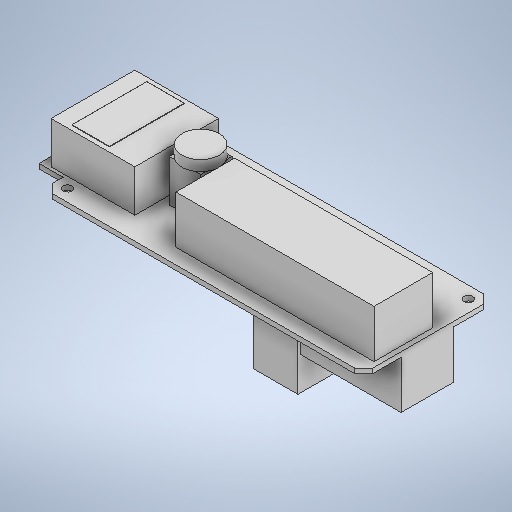
# Autodesk Inventor part: teaser_PCB
Saved by Autodesk Inventor 2025.2 (Build 292293000, 293)
## iProperties
Created: 2025-03-24
Part Number: teaser_PCB
Material: Generic
Document SubType Name: Modeling
Designer: Acer
Density: 1 g/cm^3
Appearance: Default
Author: Acer
Autodesk Inventor part; units mm, degrees
ref_plane "YZ Plane" through (0, 0, 0) normal (1, 0, 0) x (0, 1, 0)
ref_plane "XZ Plane" through (0, 0, 0) normal (0, 1, 0) x (-1, 0, 0)
ref_plane "XY Plane" through (0, 0, 0) normal (0, 0, 1) x (1, 0, 0)
sketch "Sketch1" plane through (0, 0, 0) normal (0, 1, 0) x (-1, 0, 0)
  line L0 (-57.5, 21.5) -> (57.5, 21.5)
  line L1 (57.5, 21.5) -> (57.5, -21.5)
  line L2 (57.5, -21.5) -> (-57.5, -21.5)
  line L3 (-57.5, -21.5) -> (-57.5, 21.5)
  line L4 (-57.5, 21.5) -> (57.5, -21.5) construction
  line L5 (57.5, 21.5) -> (-57.5, -21.5) construction
  point P0 (0, 0)
  dimension "d0" = 115
  dimension "d1" = 43
  constraints: 12 end point, 2 midpoint, 2 parallel, 1 horizontal, 1 perpendicular
  measures "d0" distance of L1.end L2.end
  measures "d1" distance of L0.end L1.end
extrude "Extrusion1" add sketch "Sketch1" along normal blind 1.6
sketch "Sketch2" plane through (0, 1.6, 0) normal (0, 1, 0) x (1, 0, 0)
  line L0 (57.5, 21.5) -> (-57.5, 21.5) projected
  line L1 (57.5, 21.5) -> (54.5, 21.5)
  line L2 (57.5, -21.5) -> (57.5, 21.5) projected
  line L3 (54.5, 21.5) -> (57.5, 21.5)
  line L4 (57.5, 21.5) -> (57.5, 18.5)
  line L5 (57.5, 18.5) -> (54.5, 21.5)
  point P0 (0, 0)
  dimension "d4" = 3
  dimension "d5" = 3
  constraints: 8 end point, 2 point on line, 1 perpendicular
  measures "d4" distance of L0.start L1.end
  measures "d5" distance of L0.start L4.end
extrude "Extrusion2" cut sketch "Sketch2" against normal blind 1.6
sketch "Sketch3" plane through (0, 1.6, 0) normal (0, 1, 0) x (1, 0, 0)
  line L0 (57.5, -21.5) -> (57.5, 18.5) projected
  circle A0 centre (53.5, 17.5) radius 1.5
  point P0 (0, 0)
  dimension "d11" = 3
  constraints: 1 centre point
  measures "d11" diameter of A0
extrude "Extrusion3" cut sketch "Sketch3" against normal blind 1.6
sketch "Sketch4" plane through (0, 1.6, 0) normal (0, 1, 0) x (1, 0, 0)
  line L0 (-57.5, 21.5) -> (-57.5, -21.5) projected
  line L1 (-57.5, 15) -> (-49.5, 15)
  line L2 (-49.5, 15) -> (-49.5, 18.5)
  line L3 (54.5, 21.5) -> (-57.5, 21.5) projected
  line L4 (-46.5, 21.5) -> (-49.5, 18.5)
  circle A0 centre (-45.5, 18) radius 1.5
  point P0 (0, 0)
  dimension "d15" = 8
  dimension "d16" = 3.5
  dimension "d20" = 3
  constraints: 6 end point, 1 centre point, 1 perpendicular, 1 point on line
  measures "d15" distance of L1.start L1.end
  measures "d16" distance of L1.end L2.end
  measures "d20" diameter of A0
extrude "Extrusion4" cut sketch "Sketch4" against normal blind 1.6 contours L3 L4 L2 L1 L0
sketch "Sketch5" plane through (0, 1.6, 0) normal (0, 1, 0) x (1, 0, 0)
  line L0 (54.5, 21.5) -> (-46.5, 21.5) projected
  circle A0 centre (-45.5, 17.5) radius 1.5
  point P0 (0, 0)
  dimension "d25" = 3
  constraints: 1 centre point
  measures "d25" diameter of A0
extrude "Extrusion5" cut sketch "Sketch5" against normal blind 1.6
mirror "Mirror1" about plane through (0, 0, 0) normal (0, 0, 1) of "Extrusion4", "Extrusion5", "Extrusion2"
sketch "Sketch7" plane through (0, 1.6, 0) normal (0, 1, 0) x (1, 0, 0)
  line L0 (-54.4988, 14.0073) -> (-26.4988, 14.0073)
  line L1 (-26.4988, 14.0073) -> (-26.4988, -13.9927)
  line L2 (-26.4988, -13.9927) -> (-54.4988, -13.9927)
  line L3 (-54.4988, -13.9927) -> (-54.4988, 14.0073)
  point P0 (0, 0)
  dimension "d30" = 28
  dimension "d31" = 28
  constraints: 8 end point, 2 parallel, 1 horizontal, 1 perpendicular
  measures "d30" distance of L1.end L2.end
  measures "d31" distance of L0.end L1.end
extrude "Extrusion6" add sketch "Sketch7" along normal blind 14
sketch "Sketch8" plane through (0, 15.6, 0) normal (0, 1, 0) x (1, 0, 0)
  line L0 (-26.4988, 14.0073) -> (-26.4988, -13.9927) projected
  line L1 (-26.4988, 14.0073) -> (-36.4988, 14.0073)
  line L2 (-54.4988, 14.0073) -> (-26.4988, 14.0073) projected
  line L3 (-36.4988, 14.0073) -> (-37.9988, 14.0073)
  line L4 (-37.9988, 14.0073) -> (-36.4988, 14.0073)
  line L5 (-36.4988, 14.0073) -> (-36.4988, 12.5073)
  line L6 (-36.4988, 12.5073) -> (-48.9988, 12.5073)
  line L7 (-48.9988, 12.5073) -> (-48.9988, -12.4927)
  line L8 (-48.9988, -12.4927) -> (-36.4988, -12.4927)
  line L9 (-36.4988, -12.4927) -> (-36.4988, 12.5073)
  point P0 (0, 0)
  dimension "d34" = 10
  dimension "d35" = 1.5
  dimension "d36" = 1.5
  dimension "d37" = 12.5
  dimension "d38" = 25
  constraints: 16 end point, 3 equal length, 2 perpendicular, 2 point on line, 1 horizontal
  measures "d34" distance of L0.start L1.end
  measures "d35" distance of L1.end L3.end
  measures "d36" distance of L1.end L5.end
  measures "d37" distance of L8.end L7.end
  measures "d38" distance of L7.end L6.end
extrude "Extrusion7" add sketch "Sketch8" along normal blind 0.2
sketch "Sketch9" plane through (0, 1.6, 0) normal (0, 1, 0) x (1, 0, 0)
  line L0 (-57.5, 15) -> (-57.5, -15) projected
  line L1 (-57.5, 15) -> (-23.75, 15)
  line L2 (-23.75, 15) -> (-23.75, 5.25)
  line L3 (-23.75, 5.25) -> (-13.25, 5.25)
  line L4 (-13.25, 5.25) -> (-13.25, -5.25)
  line L5 (-13.25, -5.25) -> (-23.75, -5.25)
  line L6 (-23.75, -5.25) -> (-23.75, 5.25)
  point P0 (0, 0)
  dimension "d41" = 33.75
  dimension "d43" = 9.75
  dimension "d44" = 10.5
  dimension "d45" = 10.5
  constraints: 12 end point, 2 horizontal, 2 parallel, 1 perpendicular, 1 vertical
  measures "d41" distance of L0.start L1.end
  measures "d43" distance of L1.end L2.end
  measures "d44" distance of L4.end L5.end
  measures "d45" distance of L3.end L4.end
extrude "Extrusion8" add sketch "Sketch9" along normal blind 14
sketch "Sketch10" plane through (0, 15.6, 0) normal (0, 1, 0) x (1, 0, 0)
  circle A0 centre (-18.5, 0) radius 6.25
  point P0 (0, 0)
  dimension "d48" = 12.5
  constraints: 1 centre point
  measures "d48" diameter of A0
extrude "Extrusion9" add sketch "Sketch10" along normal blind 3.5
sketch "Sketch11" plane through (0, 1.6, 0) normal (0, 1, 0) x (1, 0, 0)
  line L0 (54.5, -21.5) -> (57.5, -18.5) projected
  line L1 (57.5, -18.5) -> (55.85, -18.5)
  line L2 (55.85, -18.5) -> (55.85, -16.4)
  line L3 (55.85, -16.4) -> (57.5, -16.4)
  line L4 (57.5, -16.4) -> (57.5, -18.5)
  line L5 (55.85, -16.4) -> (-10.35, -16.4)
  line L6 (-10.35, -16.4) -> (-10.35, 3.2)
  line L7 (-10.35, 3.2) -> (55.85, 3.2)
  line L8 (55.85, 3.2) -> (55.85, -16.4)
  point P0 (0, 0)
  dimension "d51" = 1.65
  dimension "d52" = 2.1
  dimension "d53" = 66.2
  dimension "d54" = 19.6
  constraints: 16 end point, 4 parallel, 2 horizontal, 2 perpendicular
  measures "d51" distance of L2.end L3.end
  measures "d52" distance of L1.end L2.end
  measures "d53" distance of L6.end L7.end
  measures "d54" distance of L5.end L6.end
extrude "Extrusion10" add sketch "Sketch11" along normal blind 16 contours L5 L6 L7 L8
sketch "Sketch12" plane through (0, 0, 0) normal (0, -1, 0) x (1, 0, 0)
  line L0 (57.5, 18.5) -> (57.5, -18.5) projected
  line L1 (57.5, -18.5) -> (57.5, -8.5)
  line L2 (57.5, -8.5) -> (48.2, -8.5)
  line L3 (48.2, -8.5) -> (48.2, 9)
  line L4 (48.2, 9) -> (57.5, 9)
  line L5 (57.5, 9) -> (57.5, -8.5)
  point P0 (0, 0)
  dimension "d57" = 10
  dimension "d58" = 9.3
  dimension "d59" = 17.5
  constraints: 10 end point, 2 parallel, 1 horizontal, 1 perpendicular, 1 point on line
  measures "d57" distance of L0.end L1.end
  measures "d58" distance of L3.end L4.end
  measures "d59" distance of L2.end L3.end
extrude "Extrusion11" add sketch "Sketch12" along normal blind 16
sketch "Sketch13" plane through (0, 0, 0) normal (0, -1, 0) x (1, 0, 0)
  line L0 (57.5, -8.5) -> (48.2, -8.5) projected
  line L1 (48.2, -8.5) -> (48.2, -16)
  line L2 (48.2, -16) -> (24, -16)
  line L3 (24, -16) -> (24, 9)
  line L4 (24, 9) -> (48.2, 9)
  line L5 (48.2, 9) -> (48.2, -16)
  line L6 (24, -16) -> (24, -20)
  line L7 (54.5, -21.5) -> (-46.5, -21.5) projected
  line L8 (24, -20) -> (9, -20)
  line L9 (24, 9) -> (24, 10)
  line L10 (24, 10) -> (9, 10)
  line L11 (9, 10) -> (9, -20)
  line L12 (9, -20) -> (24, -20)
  line L13 (24, -20) -> (24, 10)
  point P0 (0, 0)
  dimension "d62" = 7.5
  dimension "d63" = 24.2
  dimension "d64" = 25
  dimension "d65" = 4
  dimension "d66" = 15
  dimension "d67" = 1
  constraints: 24 end point, 4 parallel, 4 perpendicular, 2 horizontal, 2 vertical
  measures "d62" distance of L0.end L1.end
  measures "d63" distance of L3.end L4.end
  measures "d64" distance of L2.end L3.end
  measures "d65" distance of L2.end L6.end
  measures "d66" distance of L6.end L8.end
  measures "d67" distance of L3.end L9.end
extrude "Extrusion12" add sketch "Sketch13" along normal blind 16 contours L1 L2 L3 L4 L5
sketch "Sketch14" plane through (0, 0, 0) normal (0, -1, 0) x (1, 0, 0)
  line L0 (24, -16) -> (24, 9) projected
  line L1 (24, -16) -> (24, -20)
  line L2 (24, -20) -> (9, -20)
  line L3 (24, 9) -> (24, 10)
  line L4 (24, 10) -> (9, 10)
  line L5 (9, 10) -> (9, -20)
  line L6 (9, -20) -> (24, -20)
  line L7 (24, -20) -> (24, 10)
  point P0 (0, 0)
  dimension "d70" = 4
  dimension "d71" = 15
  dimension "d72" = 1
  constraints: 14 end point, 2 parallel, 2 perpendicular, 2 vertical, 1 horizontal
  measures "d70" distance of L0.start L1.end
  measures "d71" distance of L1.end L2.end
  measures "d72" distance of L0.end L3.end
extrude "Extrusion13" add sketch "Sketch14" along normal blind 27
body "Solid1"
